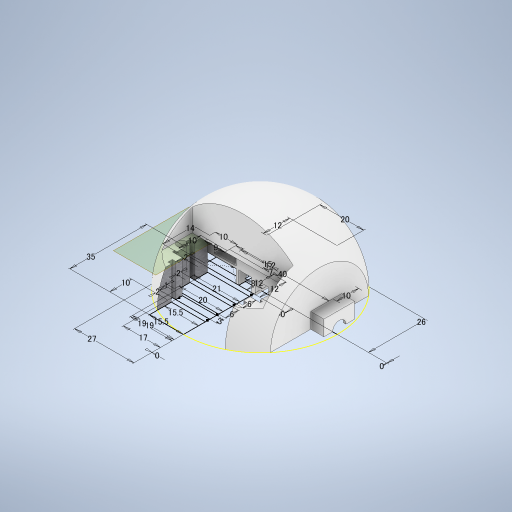
# Autodesk Inventor part: naibu
Saved by Autodesk Inventor 2023 (Build 270158000, 158)
## iProperties
Created: 2022-10-08
Part Number: naibu
Material: ABS プラスチック
Document SubType Name: Modeling
Designer: ellie
Density: 1.06 g/cm^3
Appearance: 積雪
Author: ellie
Autodesk Inventor part; units mm, degrees
ref_plane "YZ Plane" through (0, 0, 0) normal (1, 0, 0) x (0, 1, 0)
ref_plane "XZ Plane" through (0, 0, 0) normal (0, 1, 0) x (-1, 0, 0)
ref_plane "XY Plane" through (0, 0, 0) normal (0, 0, 1) x (1, 0, 0)
sketch "スケッチ1" plane through (0, 0, 0) normal (0, 1, 0) x (-1, 0, 0)
  circle A0 centre (0, 0) radius 35
  line L0 (0, 0) -> (0, -35)
  line L1 (0, 0) -> (0, 35)
  dimension "d0" = 70
  constraints: 4 end point, 2 point on circle, 2 vertical, 1 centre point, 1 coincident
  measures "d0" diameter of A0
revolve "回転1" add sketch "スケッチ1" angle 180 about axis through (0, 0, 0) along (0, 0, 1) picked at (-2.5961, -23.0408) contours L1 L0 A0
sketch "スケッチ5" plane through (0, 0, 0) normal (0, -1, 0) x (1, 0, 0)
  line L0 (-20, -23) -> (20, -23)
  line L1 (20, -23) -> (20, -13)
  line L2 (20, -13) -> (-20, -13)
  line L3 (-20, -13) -> (-20, -23)
  line L4 (-20, -15) -> (-20, -13)
  line L5 (0, 25) -> (-17, 25)
  line L6 (-17, 25) -> (-17, 23)
  line L7 (-17, 23) -> (0, 23)
  line L8 (0, 23) -> (0, 25)
  line L9 (0, 20) -> (-20, 20)
  line L10 (-20, 20) -> (-20, 19)
  line L11 (-20, 19) -> (0, 19)
  line L12 (0, 19) -> (0, 20)
  line L13 (0, 13) -> (-21, 13)
  line L14 (-21, 13) -> (-21, 11)
  line L15 (-21, 11) -> (0, 11)
  line L16 (0, 11) -> (0, 13)
  line L17 (0, 5) -> (-23, 5)
  line L18 (-23, 5) -> (-23, 3)
  line L19 (-23, 3) -> (0, 3)
  line L20 (0, 3) -> (0, 5)
  circle A0 centre (0, 0) radius 35 projected
  circle A1 centre (0, 0) radius 35 projected
  line L21 (0, 35) -> (0, -35)
  line L22 (35, 0) -> (-35, 0)
  line L23 (-32, 2) -> (-23, 2)
  line L24 (-23, 2) -> (-23, -8)
  line L25 (-23, -8) -> (-32, -8)
  line L26 (-32, -8) -> (-32, 2)
  line L27 (-23, -8.0262) -> (-23, 2)
  line L28 (-27, 22.2711) -> (-27, -22.2711)
  line L29 (-15.5, 25) -> (0, 25)
  line L30 (0, 25) -> (0, 35)
  line L31 (0, 35) -> (-15.5, 35)
  line L32 (-15.5, 35) -> (-15.5, 25)
  line L33 (-15.5, 23) -> (0, 23)
  line L34 (0, 23) -> (0, 20)
  line L35 (0, 20) -> (-15.5, 20)
  line L36 (-15.5, 20) -> (-15.5, 23)
  line L37 (-19, 13) -> (0, 13)
  line L38 (0, 13) -> (0, 19)
  line L39 (0, 19) -> (-19, 19)
  line L40 (-19, 19) -> (-19, 13)
  line L41 (-19, 11) -> (0, 11)
  line L42 (0, 11) -> (0, 5)
  line L43 (0, 5) -> (-19, 5)
  line L44 (-19, 5) -> (-19, 11)
  line L45 (-23, -3) -> (-39.6865, -3)
  line L46 (-23, -3) -> (-7.8337, -3)
  line L47 (-8, 3) -> (-23, 3)
  line L48 (-23, 3) -> (-23, -9)
  line L49 (-23, -9) -> (-8, -9)
  line L50 (-8, -9) -> (-8, 3)
  line L51 (-8, 3) -> (-23, -9) construction
  line L52 (-23, 3) -> (-8, -9) construction
  line L53 (-23, 4) -> (-33, 4)
  line L54 (-33, 4) -> (-33, -10)
  line L55 (-33, -10) -> (-23, -10)
  line L56 (-23, -10) -> (-23, 4)
  line L57 (-23, 4) -> (-33, -10) construction
  line L58 (-33, 4) -> (-23, -10) construction
  line L59 (-8, 3) -> (-1, 3)
  line L60 (-1, 3) -> (-1, -9)
  line L61 (-1, -9) -> (-8, -9)
  line L62 (-8, -9) -> (-8, 3)
  line L63 (-8, 3) -> (-1, -9) construction
  line L64 (-1, 3) -> (-8, -9) construction
  line L65 (-23, 2) -> (-27, 2)
  line L66 (-23, -8) -> (-27, -8)
  line L67 (-23, 4) -> (-27, 4)
  line L68 (-23, -10) -> (-27, -10)
  line L69 (23.4307, -26) -> (-23.4307, -26)
  line L70 (-8, 3) -> (-6.8, 3)
  line L71 (-6.8, 3) -> (-6.8, -9)
  line L72 (-6.8, -9) -> (-8, -9)
  line L73 (-8, -9) -> (-8, 3)
  line L74 (-3, 5) -> (0, 5)
  line L75 (0, 20) -> (-4, 20)
  line L76 (-4, 19) -> (0, 19)
  line L77 (0, 19) -> (0, 20)
  line L78 (-6, 5) -> (-1, 5)
  line L79 (-1, 3) -> (-6, 3)
  point P0 (0, -23)
  point P1 (0, -13)
  point P2 (0, 24)
  point P3 (0, 19.5)
  point P4 (0, 12)
  point P5 (0, 4)
  point P6 (-20, -18)
  point P7 (-27, -0.5262)
  point P8 (-27, -8)
  point P9 (-15.5, 21.5)
  point P10 (-15.5, 31.3807)
  point P11 (0, 25)
  point P12 (0, 23)
  point P13 (0, 11)
  point P14 (0, 13)
  point P15 (-27, 0)
  point P16 (-32, 0)
  point P17 (-23, 0)
  point P18 (-15.5, -3)
  point P19 (-28, -3)
  point P20 (-4.5, -3)
  point P21 (-8, -9)
  point P22 (-8, 3)
  point P23 (-27, 0.5)
  point P24 (-28, 0.4738)
  point P25 (-28, -11.5262)
  point P26 (-27, -11.5)
  point P27 (-23, 2)
  point P28 (-23, 2)
  point P29 (-8, 0)
  point P30 (-1, 0)
  point P31 (0, 19)
  point P32 (0, 20)
  point P33 (-27, -10)
  point P34 (-27, 4)
  dimension "d12" = 40
  dimension "d13" = 10
  dimension "d23" = 17
  dimension "d24" = 2
  dimension "d27" = 20
  dimension "d28" = 1
  dimension "d30" = 21
  dimension "d31" = 2
  dimension "d33" = 2
  dimension "d88" = 0
  dimension "d89" = 0
  dimension "d90" = 12
  dimension "d92" = 20
  dimension "d93" = 10
  dimension "d97" = 9
  dimension "d98" = 10
  dimension "d113" = 27
  dimension "d122" = 15.5
  dimension "d123" = 35
  dimension "d124" = 3
  dimension "d125" = 15.5
  dimension "d126" = 6
  dimension "d127" = 6
  dimension "d128" = 19
  dimension "d129" = 19
  dimension "d147" = 12
  dimension "d149" = 8
  dimension "d151" = 15
  dimension "d161" = 14
  dimension "d162" = 10
  dimension "d164" = 12
  dimension "d165" = 7
  dimension "d170" = 26
  dimension "d175" = 1.2
  dimension "d207" = 0
  constraints: 158 end point, 31 parallel, 20 horizontal, 17 perpendicular, 16 point on line, 15 midpoint, 10 collinear, 1 vertical, 20 other
  measures "d12" distance of L2.end L1.end
  measures "d13" distance of L1.end L0.end
  measures "d23" distance of L7.end L6.end
  measures "d24" distance of L6.end L5.end
  measures "d27" distance of L11.end L10.end
  measures "d28" distance of L10.end L9.end
  measures "d30" distance of L15.end L14.end
  measures "d31" distance of L14.end L13.end
  measures "d33" distance of L18.end L17.end
  measures "d89" distance from line of point (0, 0) L22
  measures "d90" distance from line of L0 point (0, -35)
  measures "d92" distance of the line from the sketch origin of L3
  measures "d93" distance from line of L5 point (0, 35)
  measures "d97" distance of L24.end L25.end
  measures "d98" distance of L23.end L24.end
  measures "d113" distance of the line from the sketch origin of L28
  measures "d122" distance of the line from the sketch origin of L32
  measures "d123" distance between parallel lines of L31 L22
  measures "d124" distance of L33.end L34.end
  measures "d126" distance of L38.end L37.end
  measures "d127" distance of L41.end L42.end
  measures "d128" distance of the line from the sketch origin of L44
  measures "d129" distance of the line from the sketch origin of L40
  measures "d147" distance of L48.end L47.end
  measures "d149" distance of the line from the sketch origin of L50
  measures "d151" distance between parallel lines of L50 L24
  measures "d161" distance between parallel lines of L55 L53
  measures "d162" distance between parallel lines of L48 L54
  measures "d164" distance between parallel lines of L61 L59
  measures "d165" distance between parallel lines of L50 L60
  measures "d170" distance between parallel lines of L69 L22
  measures "d175" distance of L71.end L72.end
  measures "d207" distance between parallel lines of L47 L19
extrude "GNSボード" cut sketch "スケッチ5" against normal blind 16 contours L8 L7 L6 L5
extrude "GNSボード止めるよう" cut sketch "スケッチ5" against normal blind 15 contours L21 L5 L32 A0 | L21 L9 L36 L7
extrude "アルミ板１" cut sketch "スケッチ5" against normal blind 20 contours L11 L10 L9 L12
extrude "メイン基板" cut sketch "スケッチ5" against normal blind 17.5 contours L15 L14 L13 L16
extrude "メイン止めるよう" cut sketch "スケッチ5" against normal blind 15 contours L17 L44 L15 L21 | L13 L40 L11 L21
extrude "アルミ板２" cut sketch "スケッチ5" against normal blind 20 contours L19 L18 L17 L20
extrude "電池ボックス入れ" cut sketch "スケッチ5" against normal blind 13 contours L3 L2 L21 L0 | L21 L2 L1 L0
extrude "side ut" cut sketch "スケッチ5" against normal blind 100 contours A0 L45 L54 L55 L28 | A0 L22 L54 L45 | L55 L54 L45 L26 L25 L28 | A0 L28 L53 L54 L22 | L54 L22 L26 L45 | L25 L26 L45 L28 | L54 L53 L28 L23 L26 L22 | L26 L22 L28 L45 | L22 L26 L23 L28
extrude "motor case" add sketch "スケッチ5" against normal blind 7 contours L55 L54 L45 L26 L25 L28 | L28 L25 L27 L48 L56 L55 | L50 L46 L24 L22 | L22 L24 L48 L19 L50 | L54 L22 L26 L45 | L28 L45 L24 L25 | L25 L26 L45 L28 | L24 L45 L28 L22 | L22 L28 L23 L24 | L50 L49 L48 L27 L24 L46 | L54 L53 L28 L23 L26 L22 | L26 L22 L28 L45 | L53 L18 L48 L23 L28 | L22 L26 L23 L28
extrude "bottom cut" cut sketch "スケッチ5" against normal blind 90 contours L69 A0 L21 | L21 A0 L69
extrude "motor" cut sketch "スケッチ5" against normal blind 6 contours L60 L61 L71 L22 | L22 L71 L19 L60 | L71 L61 L50 L22 | L22 L50 L19 L71 | L50 L46 L24 L22 | L22 L24 L48 L19 L50 | L28 L45 L24 L25 | L25 L26 L45 L28 | L24 L45 L28 L22 | L22 L28 L23 L24 | L50 L49 L48 L27 L24 L46 | L26 L22 L28 L45 | L22 L26 L23 L28
extrude "motor block" add sketch "スケッチ5" against normal blind 10 contours L71 L61 L50 L22 | L22 L50 L19 L71
sketch "スケッチ27" plane through (-33, 0, -10) normal (-1, 0, 0) x (0, 0, 1)
  line L0 (14, 0) -> (0, 0) projected
  circle A0 centre (7, 0) radius 3
  point P0 (10, 0)
  dimension "d198" = 6
  constraints: 1 centre point, 1 midpoint
  measures "d198" diameter of A0
extrude "moter shaft" cut sketch "スケッチ27" against normal blind 27
mirror "ミラー13" about plane through (0, 0, 0) normal (1, 0, 0) of "メイン止めるよう", "メイン基板", "アルミ板１", "GNSボード止めるよう", "GNSボード", "アルミ板２", "motor", "motor case", "moter shaft", "電池ボックス入れ", "side ut", "motor block"
ref_plane "作業平面5" through (-17, 17.5, 23) normal (0, -1, 0) x (1, 0, 0)
ref_plane "作業平面6" through (20, 13, -13) normal (0, 0, -1) x (1, 0, 0)
sketch "スケッチ38" plane through (20, 13, -13) normal (0, 0, -1) x (1, 0, 0)
  line L0 (-40, 13) -> (0, 13) projected
  line L1 (-40, 13) -> (-40, 0) projected
  line L2 (-40, 0) -> (0, 0) projected
  line L3 (0, 13) -> (0, 0) projected
  line L4 (-38, 6) -> (-28, 6)
  line L5 (-28, 6) -> (-28, -3)
  line L6 (-28, -3) -> (-38, -3)
  line L7 (-38, -3) -> (-38, 6)
  point P0 (-20, 13)
  dimension "d235" = 3
  dimension "d236" = 9
  dimension "d237" = 10
  dimension "d238" = 2
  constraints: 8 end point, 2 parallel, 1 horizontal, 1 perpendicular
  measures "d235" distance between parallel lines of L6 L2
  measures "d236" distance between parallel lines of L6 L4
  measures "d237" distance between parallel lines of L7 L5
  measures "d238" distance between parallel lines of L1 L7
extrude "battery wire" cut sketch "スケッチ38" against normal blind 18 contours L7 L4 L5 L2 | L2 L5 L6 L7
ref_plane "作業平面7" through (27, 35, 4) normal (0, -1, 0) x (1, 0, 0)
sketch "スケッチ41" plane through (-17, 0, 23) normal (0, -1, 0) x (1, 0, 0)
  line L0 (-16, -23) -> (-15, -23) projected
  line L1 (-15, -23) -> (-15, -21) projected
  line L2 (-15, -21) -> (-6, -21) projected
  line L3 (-6, -21) -> (-6, -18) projected
  line L4 (-6, -18) -> (-2, -18) projected
  line L5 (-2, -18) -> (-2, -12) projected
  line L6 (-2, -12) -> (-4, -12) projected
  line L7 (-4, -12) -> (-4, -10) projected
  line L8 (-4, -10) -> (-2, -10) projected
  line L9 (-2, -10) -> (-2, -4) projected
  line L10 (-2, -4) -> (-3, -4) projected
  line L11 (-3, -4) -> (-3, -3) projected
  line L12 (-3, -3) -> (1.5, -3) projected
  line L13 (1.5, -3) -> (1.5, 0) projected
  line L14 (1.5, 0) -> (0, 0) projected
  line L15 (0, 0) -> (0, 2) projected
  line L16 (0, 2) -> (1.5, 2) projected
  line L17 (1.5, 2) -> (1.5, 8.3807) projected
  arc A0 (1.5, 8.3807) -> (-10, -0.7289) centre (17, -23) ccw projected
  line L18 (-10, -0.7289) -> (-10, -19) projected
  line L19 (-10, -19) -> (-16, -19) projected
  line L20 (-16, -19) -> (-16, -23) projected
  line L21 (-2, -18) -> (-2, -12) projected
  line L22 (-4, -10) -> (-4, -12) projected
  line L23 (0, 2) -> (0, 0) projected
  circle A1 centre (-4, 0) radius 2
  dimension "d252" = 4
  dimension "d253" = 4
  dimension "d254" = 3
  constraints: 1 centre point
  measures "d252" diameter of A1
  measures "d253" distance from line of A1.centre L15
  measures "d254" distance from line of A1.centre L12
extrude "top lock 10mm" cut sketch "スケッチ41" against normal blind 10 contours A1
mirror "ミラー15" about plane through (0, 0, 0) normal (1, 0, 0) of "top lock 10mm"
sketch "スケッチ42" plane through (-33, 0, -10) normal (0, -1, 0) x (1, 0, 0)
  circle A0 centre (9.5, -8) radius 2
  line L0 (13, -13) -> (13, -3) projected
  line L1 (10, 2) -> (1, 2) projected
  point P0 (33, 10)
  dimension "d257" = 3.5
  dimension "d258" = 4
  dimension "d259" = 10
  constraints: 1 centre point
  measures "d257" distance from line of A0.centre L0
  measures "d258" diameter of A0
  measures "d259" distance from line of A0.centre L1
extrude "bottom lock" cut sketch "スケッチ42" against normal blind 10
mirror "ミラー16" about plane through (0, 0, 0) normal (1, 0, 0) of "bottom lock"
ref_plane "作業平面8" through (-17, 15, 23) normal (0, -1, 0) x (1, 0, 0)
sketch "スケッチ45" plane through (-17, 15, 23) normal (0, -1, 0) x (1, 0, 0)
  circle A0 centre (-4, 0) radius 2 projected
  line L0 (-16, -23) -> (-15, -23) projected
  line L1 (-15, -23) -> (-15, -21) projected
  line L2 (-15, -21) -> (-6, -21) projected
  line L3 (-6, -21) -> (-6, -18) projected
  line L4 (-6, -18) -> (-2, -18) projected
  line L5 (-2, -18) -> (-2, -12) projected
  line L6 (-2, -12) -> (-4, -12) projected
  line L7 (-4, -12) -> (-4, -10) projected
  line L8 (-4, -10) -> (-2, -10) projected
  line L9 (-2, -10) -> (-2, -4) projected
  line L10 (-2, -4) -> (-3, -4) projected
  line L11 (-3, -4) -> (-3, -3) projected
  line L12 (-3, -3) -> (1.5, -3) projected
  line L13 (1.5, -3) -> (1.5, 0) projected
  line L14 (1.5, 0) -> (0, 0) projected
  line L15 (0, 0) -> (0, 2) projected
  line L16 (0, 2) -> (1.5, 2) projected
  line L17 (1.5, 2) -> (1.5, 8.3807) projected
  arc A1 (1.5, 8.3807) -> (-10, -0.7289) centre (17, -23) ccw projected
  line L18 (-10, -0.7289) -> (-10, -19) projected
  line L19 (-10, -19) -> (-16, -19) projected
  line L20 (-16, -19) -> (-16, -23) projected
  arc A2 (32.5, 4.5636) -> (1.5, 4.5636) centre (17, -23) ccw projected
  line L21 (1.5, 2) -> (1.5, 4.5636) projected
  line L22 (32.5, 2) -> (1.5, 2) projected
  line L23 (32.5, 2) -> (32.5, 4.5636) projected
  circle A3 centre (38, 0) radius 2 projected
  line L24 (49, -23) -> (50, -23) projected
  line L25 (50, -19) -> (50, -23) projected
  line L26 (44, -19) -> (50, -19) projected
  line L27 (44, -19) -> (44, -0.7289) projected
  arc A4 (44, -0.7289) -> (32.5, 8.3807) centre (17, -23) ccw projected
  line L28 (32.5, 8.3807) -> (32.5, 2) projected
  line L29 (32.5, 2) -> (34, 2) projected
  line L30 (34, 2) -> (34, 0) projected
  line L31 (34, 0) -> (32.5, 0) projected
  line L32 (32.5, 0) -> (32.5, -3) projected
  line L33 (32.5, -3) -> (37, -3) projected
  line L34 (37, -3) -> (37, -4) projected
  line L35 (37, -4) -> (36, -4) projected
  line L36 (36, -4) -> (36, -10) projected
  line L37 (36, -10) -> (38, -10) projected
  line L38 (38, -10) -> (38, -12) projected
  line L39 (38, -12) -> (36, -12) projected
  line L40 (36, -12) -> (36, -18) projected
  line L41 (36, -18) -> (40, -18) projected
  line L42 (40, -18) -> (40, -21) projected
  line L43 (40, -21) -> (49, -21) projected
  line L44 (49, -21) -> (49, -23) projected
  circle A5 centre (38, 0) radius 2 projected
  circle A6 centre (-4, 0) radius 2 projected
  line L45 (34, 0) -> (0, 0) projected
  line L46 (34, 0) -> (34, 2) projected
  line L47 (34, 2) -> (0, 2) projected
  line L48 (0, 0) -> (0, 2) projected
  line L49 (32.5, -3) -> (1.5, -3) projected
  line L50 (32.5, -3) -> (32.5, 0) projected
  line L51 (1.5, 0) -> (32.5, 0) projected
  line L52 (1.5, -3) -> (1.5, 0) projected
  line L53 (-2, -4) -> (36, -4) projected
  circle A7 centre (38, 0) radius 2 projected
  line L54 (36, -10) -> (-2, -10) projected
  line L55 (36, -10) -> (36, -4) projected
  line L56 (-2, -4) -> (36, -4) projected
  line L57 (-2, -10) -> (-2, -4) projected
  line L58 (-2, -12) -> (36, -12) projected
  line L59 (36, -18) -> (-2, -18) projected
  line L60 (36, -18) -> (36, -12) projected
  line L61 (-2, -12) -> (36, -12) projected
  line L62 (-2, -18) -> (-2, -12) projected
  line L63 (40, -20) -> (-6, -20) projected
  line L64 (40, -20) -> (40, -18) projected
  line L65 (40, -18) -> (-6, -18) projected
  line L66 (-6, -20) -> (-6, -18) projected
  line L67 (9, -32) -> (9, -20) projected
  line L68 (-6, -20) -> (9, -20) projected
  line L69 (-6, -21) -> (-6, -20) projected
  line L70 (-15, -21) -> (-6, -21) projected
  line L71 (-15, -31) -> (-15, -21) projected
  line L72 (-6, -31) -> (-15, -31) projected
  line L73 (-6, -32) -> (-6, -31) projected
  line L74 (9, -32) -> (-6, -32) projected
  circle A8 centre (40.5, -41) radius 2 projected
  circle A9 centre (-6.5, -41) radius 2 projected
  line L75 (25, -29) -> (23.8, -29) projected
  line L76 (23.8, -32) -> (23.8, -29) projected
  line L77 (23.8, -32) -> (18, -32) projected
  line L78 (18, -32) -> (18, -20) projected
  line L79 (18, -20) -> (16, -20) projected
  line L80 (16, -20) -> (16, -32) projected
  line L81 (16, -32) -> (10.2, -32) projected
  line L82 (10.2, -32) -> (10.2, -29) projected
  line L83 (10.2, -29) -> (9, -29) projected
  line L84 (9, -29) -> (9, -32) projected
  line L85 (9, -32) -> (-6, -32) projected
  line L86 (-6, -32) -> (-6, -31) projected
  line L87 (-6, -31) -> (-15, -31) projected
  line L88 (-15, -31) -> (-15, -29) projected
  line L89 (-15, -29) -> (-16, -29) projected
  line L90 (-16, -29) -> (-16, -33) projected
  line L91 (-16, -33) -> (-10, -33) projected
  line L92 (-10, -33) -> (-10, -45.2711) projected
  arc A10 (-10, -45.2711) -> (-6.4307, -49) centre (17, -23) ccw projected
  line L93 (-6.4307, -49) -> (40.4307, -49) projected
  arc A11 (40.4307, -49) -> (44, -45.2711) centre (17, -23) ccw projected
  line L94 (44, -45.2711) -> (44, -33) projected
  line L95 (50, -33) -> (44, -33) projected
  line L96 (50, -29) -> (50, -33) projected
  line L97 (50, -29) -> (49, -29) projected
  line L98 (49, -29) -> (49, -31) projected
  line L99 (49, -31) -> (40, -31) projected
  line L100 (40, -31) -> (40, -32) projected
  line L101 (40, -32) -> (25, -32) projected
  line L102 (25, -29) -> (25, -32) projected
  line L103 (-3, -36) -> (37, -36) projected
  line L104 (37, -36) -> (37, -46) projected
  line L105 (37, -46) -> (-3, -46) projected
  line L106 (-3, -46) -> (-3, -36) projected
  line L107 (-6, -15) -> (40, -15)
  line L108 (40, -15) -> (40, 8.6228)
  line L109 (40, 8.6228) -> (-6, 8.6228)
  line L110 (-6, 8.6228) -> (-6, -15)
  dimension "d269" = 3
  constraints: 8 end point, 2 collinear, 2 parallel, 1 horizontal, 1 perpendicular, 1 tangent
  measures "d269" distance between parallel lines of L107 L65
extrude "back cut" cut sketch "スケッチ45" against normal blind 20 contours A0 | L110 A1 L17 L16 L15 L14 L13 L12 L11 L10 L9 L8 L7 L6 L5 L107 | L110 L109 A2 L17 A1 | L5 L58 L40 L107 | A2 L23 L22 L17 | L109 L108 A4 L28 A2 | L6 L7 L8 L54 L37 L38 L39 L58 | A3 | L40 L39 L38 L37 L36 L35 L34 L33 L32 L31 L30 L29 L23 L28 A4 L108 L107 | L22 L29 L30 L31 L45 L14 L15 L16 | L9 L53 L36 L54 | L45 L32 L49 L13 | L10 L11 L12 L49 L33 L34 L35 L53
sketch "スケッチ47" plane through (-23, 15, 8) normal (0, 0, 1) x (1, 0, 0)
  arc A0 (50, 7.2711) -> (-4, 7.2711) centre (23, -15) ccw projected
  arc A1 (46, 10.1396) -> (0, 10.1396) centre (23, -15) ccw projected
  arc A2 (46, 10.1396) -> (0, 10.1396) centre (23, -15) ccw projected
  line L0 (0, 0) -> (0, 10.1396) projected
  line L1 (0, 0) -> (4, 0) projected
  line L2 (42, 0) -> (4, 0) projected
  line L3 (42, 0) -> (46, 0) projected
  line L4 (46, 0) -> (46, 10.1396) projected
  line L5 (46, 0) -> (38.5, 0) projected
  line L6 (38.5, 0) -> (38.5, -15) projected
  line L7 (38.5, -15) -> (50, -15) projected
  line L8 (50, -15) -> (50, -15) projected
  line L9 (50, -15) -> (46.4307, -15) projected
  arc A3 (46.4307, -15) -> (-0.4307, -15) centre (23, -15) ccw projected
  line L10 (-0.4307, -15) -> (-4, -15) projected
  line L11 (-4, -15) -> (-4, -15) projected
  line L12 (-4, -15) -> (7.5, -15) projected
  line L13 (7.5, -15) -> (7.5, 0) projected
  line L14 (7.5, 0) -> (0, 0) projected
  line L15 (0, 0) -> (0, 10.1396) projected
  arc A4 (46, 10.1396) -> (0, 10.1396) centre (23, -15) ccw projected
  line L16 (46, 10.1396) -> (46, 0) projected
  line L17 (69.2, 0) -> (-23.2, 0) projected
  line L18 (0, 0) -> (5, 0)
  line L19 (5, 0) -> (5, 20)
  line L20 (5, 20) -> (0, 20)
  line L21 (0, 20) -> (0, 0)
  line L22 (23, 19.0735) -> (23, -15)
  line L23 (20.5, 20) -> (25.5, 20)
  line L24 (25.5, 20) -> (25.5, 0)
  line L25 (25.5, 0) -> (20.5, 0)
  line L26 (20.5, 0) -> (20.5, 20)
  line L27 (46, 0) -> (41, 0)
  line L28 (41, 0) -> (41, 20)
  line L29 (41, 20) -> (46, 20)
  line L30 (46, 20) -> (46, 0)
  point P0 (20.5, 19.9106)
  point P1 (5, 15.0167)
  point P2 (5, 0)
  point P3 (20.5, 0)
  point P4 (41, 15.0167)
  point P5 (25.5, 19.9106)
  point P6 (25.5, 0)
  point P7 (41, 0)
  dimension "d277" = 5
  dimension "d278" = 2.5
  constraints: 26 end point, 6 parallel, 4 equal length, 3 horizontal, 3 perpendicular, 2 tangent, 1 point on circle, 1 vertical, 1 other
  measures "d277" distance between parallel lines of L21 L19
  measures "d278" distance between parallel lines of L26 L22
extrude "lock rench" [suppressed]
sketch "スケッチ48" plane through (-17, 15, 23) normal (0, 1, 0) x (1, 0, 0)
  line L0 (-2, 15) -> (-2, 12) projected
  line L1 (-6, 15) -> (-2, 15) projected
  line L2 (-6, 1.2975) -> (-6, 15) projected
  arc A0 (-6, 1.2975) -> (1.5, -4.5636) centre (17, 23) ccw projected
  line L3 (1.5, -2) -> (1.5, -4.5636) projected
  line L4 (0, -2) -> (1.5, -2) projected
  line L5 (0, 0) -> (0, -2) projected
  line L6 (1.5, 0) -> (0, 0) projected
  line L7 (1.5, 3) -> (1.5, 0) projected
  line L8 (-3, 3) -> (1.5, 3) projected
  line L9 (-3, 4) -> (-3, 3) projected
  line L10 (-2, 4) -> (-3, 4) projected
  line L11 (-2, 10) -> (-2, 4) projected
  line L12 (-4, 10) -> (-2, 10) projected
  line L13 (-4, 12) -> (-4, 10) projected
  line L14 (-2, 12) -> (-4, 12) projected
  line L15 (-6, 15) -> (40, 15) projected
  line L16 (40, 15) -> (40, 1.2975) projected
  arc A1 (32.5, -4.5636) -> (40, 1.2975) centre (17, 23) ccw projected
  line L17 (32.5, -4.5636) -> (32.5, -8.3807) projected
  arc A2 (32.5, -8.3807) -> (44, 0.7289) centre (17, 23) ccw projected
  line L18 (44, 0.7289) -> (44, 45.2711) projected
  arc A3 (44, 45.2711) -> (40.4307, 49) centre (17, 23) ccw projected
  line L19 (40.4307, 49) -> (-6.4307, 49) projected
  arc A4 (-6.4307, 49) -> (-10, 45.2711) centre (17, 23) ccw projected
  line L20 (-10, 45.2711) -> (-10, 0.7289) projected
  arc A5 (-10, 0.7289) -> (1.5, -8.3807) centre (17, 23) ccw projected
  line L21 (1.5, -8.3807) -> (1.5, -4.5636) projected
  arc A6 (-6, 1.2975) -> (1.5, -4.5636) centre (17, 23) ccw projected
  line L22 (-6, 1.2975) -> (-6, 15) projected
  line L23 (36, 15) -> (36, 12) projected
  line L24 (38, 12) -> (36, 12) projected
  line L25 (38, 10) -> (38, 12) projected
  line L26 (36, 10) -> (38, 10) projected
  line L27 (36, 10) -> (36, 4) projected
  line L28 (37, 4) -> (36, 4) projected
  line L29 (37, 3) -> (37, 4) projected
  line L30 (32.5, 3) -> (37, 3) projected
  line L31 (32.5, 3) -> (32.5, 0) projected
  line L32 (34, 0) -> (32.5, 0) projected
  line L33 (34, -2) -> (34, 0) projected
  line L34 (32.5, -2) -> (34, -2) projected
  line L35 (32.5, -2) -> (32.5, -4.5636) projected
  arc A7 (32.5, -4.5636) -> (40, 1.2975) centre (17, 23) ccw projected
  line L36 (40, 15) -> (40, 1.2975) projected
  line L37 (-6, 15) -> (-2, 15) projected
  line L38 (-2, 4) -> (-6, 10)
  line L39 (-2, 10) -> (-6, 6.5714)
  circle A8 centre (-4, 8.2857) radius 2
  line L40 (-2, 4) -> (-6, 4)
  line L41 (-6, 4) -> (-6, 10)
  line L42 (-6, 10) -> (-2, 10)
  line L43 (-2, 10) -> (-2, 4)
  line L44 (-2, 15) -> (-2, 12) projected
  line L45 (-6, 1.2975) -> (-6, 15) projected
  arc A9 (-6, 1.2975) -> (1.5, -4.5636) centre (17, 23) ccw projected
  line L46 (1.5, -2) -> (1.5, -4.5636) projected
  line L47 (0, -2) -> (1.5, -2) projected
  line L48 (0, 0) -> (0, -2) projected
  line L49 (1.5, 0) -> (0, 0) projected
  line L50 (1.5, 3) -> (1.5, 0) projected
  line L51 (-3, 3) -> (1.5, 3) projected
  line L52 (-3, 4) -> (-3, 3) projected
  line L53 (-2, 4) -> (-3, 4) projected
  line L54 (-2, 10) -> (-2, 4) projected
  line L55 (-4, 10) -> (-2, 10) projected
  line L56 (-4, 12) -> (-4, 10) projected
  line L57 (-2, 12) -> (-4, 12) projected
  line L58 (36, 15) -> (40, 15) projected
  line L59 (36, 15) -> (36, 12) projected
  line L60 (38, 12) -> (36, 12) projected
  line L61 (38, 10) -> (38, 12) projected
  line L62 (36, 10) -> (38, 10) projected
  line L63 (36, 10) -> (36, 4) projected
  line L64 (37, 4) -> (36, 4) projected
  line L65 (37, 3) -> (37, 4) projected
  line L66 (32.5, 3) -> (37, 3) projected
  line L67 (32.5, 3) -> (32.5, 0) projected
  line L68 (34, 0) -> (32.5, 0) projected
  line L69 (34, -2) -> (34, 0) projected
  line L70 (32.5, -2) -> (34, -2) projected
  line L71 (32.5, -2) -> (32.5, -4.5636) projected
  arc A10 (32.5, -4.5636) -> (40, 1.2975) centre (17, 23) ccw projected
  line L72 (40, 15) -> (40, 1.2975) projected
  line L73 (36, 15) -> (40, 15) projected
  dimension "d281" = 4
  dimension "d282" = 6
  dimension "d283" = 130.601
  constraints: 12 end point, 2 parallel, 2 point on line, 1 centre point, 1 horizontal, 1 midpoint, 1 perpendicular
  measures "d281" diameter of A8
  measures "d282" distance between parallel lines of L40 L42
  measures "d283" angle of L11 L39
extrude "押し出し52" cut sketch "スケッチ48" against normal blind 10 contours A8 L12 L13 | L13 L42 A8 | A8 L38 L39 | A8 L42 L12 L39 L38 | L39 L38 A8 | L39 A8 L38
